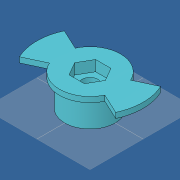
# Autodesk Inventor part: Unterdruckventil_Gegenhalter
Saved by Autodesk Inventor 2019 (Build 230136000, 136)
## iProperties
Created: 2020-09-02
Part Number: Unterdruckventil_Gegenhalter
Material: Generisch
Document SubType Name: Modeling
Designer: Stefan
Mass: 3.56095 g
Surface Area: 23.7016 cm^2
Volume: 3.56095 cm^3
Density: 1 g/cm^3
Appearance: Kadettenblau
Author: Stefan
Autodesk Inventor part; units mm, degrees
ref_plane "YZ Plane" through (0, 0, 0) normal (1, 0, 0) x (0, 1, 0)
ref_plane "XZ Plane" through (0, 0, 0) normal (0, 1, 0) x (-1, 0, 0)
ref_plane "XY Plane" through (0, 0, 0) normal (0, 0, 1) x (1, 0, 0)
sketch "Skizze1" plane through (0, 0, 0) normal (0, 1, 0) x (-1, 0, 0)
  circle A0 centre (0, 0) radius 9.5
  circle A1 centre (0, 0) radius 11.5
  circle A2 centre (0, 0) radius 8.5
  circle A3 centre (0, 0) radius 3
  circle A4 centre (0, 0) radius 20
  line L0 (10.4225, 4.8601) -> (18.1262, 8.4524)
  line L1 (10.4225, -4.8601) -> (18.1262, -8.4524)
  line L2 (28, 0) -> (-28, 0) projected
  line L3 (-10.4225, 4.8601) -> (-18.1262, 8.4524)
  line L4 (-10.4225, -4.8601) -> (-18.1262, -8.4524)
  dimension "d0" = 19
  dimension "d1" = 23
  dimension "d2" = 17
  dimension "d3" = 6
  dimension "d8" = 40
  dimension "d10" = 50
  constraints: 8 end point, 8 point on circle, 5 centre point, 5 coincident, 2 collinear, 1 point on line, 1 other
  measures "d0" diameter of A0
  measures "d1" diameter of A1
  measures "d2" diameter of A2
  measures "d3" diameter of A3
  measures "d8" diameter of A4
  measures "d10" angle of L1 L0
extrude "Extrusion1" add sketch "Skizze1" along normal blind 2 contours L2 A2 A0 | L2 A1 A0 | A0 L2 A1 | A0 L2 A2 | L2 A4 L1 A1 | A1 L0 A4 L2 | L2 A3 A2 | A2 L2 A3 | L2 A4 L3 A1 | A1 L4 A4 L2
extrude "Extrusion2" add sketch "Skizze1" against normal blind 10 contours L2 A2 A0 | A0 L2 A2 | L2 A3 A2 | A2 L2 A3
sketch "Skizze2" plane through (0, 2, 0) normal (0, 1, 0) x (1, 0, 0)
  circle A0 centre (0, 0) radius 3 projected
  arc A1 (-18.1262, 8.4524) -> (-18.1262, -8.4524) centre (0, 0) ccw projected
  line L0 (-2.8868, 5) -> (2.8868, 5)
  line L1 (2.8868, 5) -> (5.7735, 0)
  line L2 (5.7735, 0) -> (2.8868, -5)
  line L3 (2.8868, -5) -> (-2.8868, -5)
  line L4 (-2.8868, -5) -> (-5.7735, 0)
  line L5 (-5.7735, 0) -> (-2.8868, 5)
  dimension "d11" = 10
  constraints: 12 end point, 1 coincident, 1 horizontal, 13 other
  measures "d11" distance between parallel lines of L0 L3
extrude "Extrusion3" cut sketch "Skizze2" against normal blind 4
